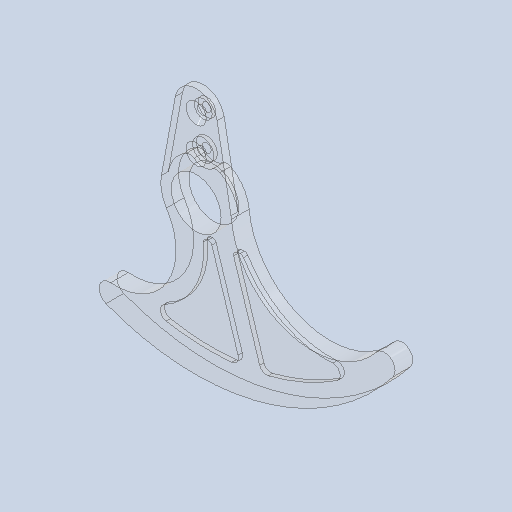
# Autodesk Inventor part: ヘッケン
Saved by Autodesk Inventor 2023 (Build 270158000, 158)
## iProperties
Created: 2022-01-09
Part Number: ヘッケン
Material: ポリカーボネート、クリア
Document SubType Name: Modeling
Designer: acps
Density: 1.2 g/cm^3
Appearance: ポリカーボネート - クリア
Mass: 12.6858 g
Surface Area: 54.0995 cm^2
Volume: 8.90232 cm^3
Author: acps
Autodesk Inventor part; units mm, degrees
ref_plane "YZ Plane" through (0, 0, 0) normal (1, 0, 0) x (0, 1, 0)
ref_plane "XZ Plane" through (0, 0, 0) normal (0, 1, 0) x (-1, 0, 0)
ref_plane "XY Plane" through (0, 0, 0) normal (0, 0, 1) x (1, 0, 0)
sketch "Sketch1" plane through (0, 0, 0) normal (0, 0, 1) x (1, 0, 0)
  line L0 (64.2929, 13) -> (99.1548, 4.0199) construction
  circle A0 centre (64.2929, 13) radius 3 construction
  circle A1 centre (64.2929, 13) radius 4.025 construction
  circle A2 centre (64.2929, 13) radius 7 construction
  arc A3 (102.6474, 8.8986) -> (63.8399, 19.9853) centre (67.7221, -39.8889) ccw construction
  circle A4 centre (99.1548, 4.0199) radius 2.5
  circle A5 centre (99.1548, 4.0199) radius 3.525
  circle A6 centre (99.1548, 4.0199) radius 6
  line L1 (64.2929, 13) -> (98.9408, 0.0186) construction
  line L2 (99.1548, 4.0199) -> (99.1548, -17.9801) construction
  line L3 (99.1548, -17.9801) -> (98.9408, 0.0186) construction
  circle A7 centre (99.1548, -17.9801) radius 10
  circle A8 centre (99.1548, -17.9801) radius 7.025
  line L4 (105.0548, 5.1108) -> (108.9881, -16.162)
  line L5 (93.2548, 5.1108) -> (89.3215, -16.162)
  line L6 (9.3628, -60) -> (214.5663, -60) construction
  arc A9 (95.4028, -0.6623) -> (65.8301, 6.1709) centre (73.5161, -27.9748) ccw construction
  line L7 (99.1548, 4.0199) -> (73.567, -55.2798) construction
  line L8 (99.1548, 4.0199) -> (154.8581, -32.5547) construction
  circle A10 centre (74.7566, -52.523) radius 3
  circle A11 centre (152.3426, -30.903) radius 3
  arc A12 (75.0109, -49.5338) -> (90.7465, -23.3931) centre (76.4523, -32.595) ccw
  arc A13 (109.1059, -16.9921) -> (149.9946, -29.0357) centre (131.9933, -14.7194) ccw
  arc A14 (73.567, -55.2798) -> (154.8581, -32.5547) centre (98.9579, 10.6509) ccw
  circle A15 centre (99.1548, -5.9801) radius 1.25
  circle A16 centre (99.1548, -5.9801) radius 3
  circle A17 centre (99.1548, -5.9801) radius 4.25
  circle A18 centre (99.1548, 4.0199) radius 1.25
  arc A19 (103.9067, -9.1813) -> (101.7399, -9.3536) centre (102.9564, -10.9411) ccw
  arc A20 (96.5698, -9.3536) -> (94.4029, -9.1813) centre (95.3533, -10.9411) ccw
  point P0 (0, 0)
  point P1 (0, 0)
  point P2 (73.6834, -55.3244)
  point P3 (154.7099, -32.7457)
  point P4 (97.1242, -8.1885)
  point P5 (102.5276, -8.5661)
  point P6 (95.7821, -8.5661)
  dimension "d19" = 6
  dimension "d20" = 6
  dimension "d0" = 36
  dimension "d1" = 8.05
  dimension "d2" = 6
  dimension "d3" = 14
  dimension "d4" = 60
  dimension "d5" = 37
  dimension "d6" = 22
  dimension "d7" = 18
  dimension "d8" = 12
  dimension "d9" = 7.05
  dimension "d10" = 20
  dimension "d11" = 14.05
  dimension "d12" = 35
  dimension "d13" = 5
  dimension "d14" = 60
  dimension "d15" = 23.34
  dimension "d17" = 66.6375
  dimension "d18" = 64.5847
  dimension "d21" = 13
  dimension "d23" = 17
  dimension "d29" = 2.5
  dimension "d30" = 6
  dimension "d31" = 8.5
  dimension "d32" = 2.5
  dimension "d43" = 10
  dimension "d44" = 2
  dimension "d45" = 2
  dimension "d46" = 56.711
  dimension "d47" = 23
  constraints: 28 point on circle, 19 centre point, 16 end point, 15 tangent, 11 coincident, 3 point on line, 1 horizontal, 1 vertical, 15 other
  measures "d0" distance of L0.start L0.end
  measures "d1" diameter of A1
  measures "d2" diameter of A0
  measures "d3" diameter of A2
  measures "d4" radius of A3
  measures "d5" distance of L3.end A1.centre
  measures "d6" distance of L2.start L2.end
  measures "d7" distance of L3.end L2.end
  measures "d8" diameter of A6
  measures "d9" diameter of A5
  measures "d10" diameter of A7
  measures "d11" diameter of A8
  measures "d12" radius of A9
  measures "d13" diameter of A4
  measures "d14" distance from line of L6 point (0, 0)
  measures "d15" angle of L2 L7
  measures "d17" distance of L2.start L8.end
  measures "d18" distance of L2.start L7.end
  measures "d21" vertical distance of point (0, 0) L0.start
  measures "d23" radius of A12
  measures "d29" diameter of A15
  measures "d30" diameter of A16
  measures "d31" diameter of A17
  measures "d32" diameter of A18
  measures "d43" distance of A17.centre L0.end
  measures "d44" radius of A19
  measures "d45" radius of A20
  measures "d46" angle of L2 L8
  measures "d47" radius of A13
extrude "Extrusion5" add sketch "Sketch1" against normal blind 5 contours A10 | A7 A20 A17 A19 | A13 A11 A14 A10 A12 A7 | A11
extrude "Extrusion6" add sketch "Sketch1" against normal blind 2 contours A5 | A6 A17 | A6 L4 A7 A17 | A17 A7 A16 A6 | A6 A17 | A6 A17 A7 L5 | A19 A17 A7 | A17 A20 A7 | A7 A16 A17
extrude "Extrusion7" add sketch "Sketch1" against normal blind 3 contours A4 | A16 A7 | A7 A16
chamfer "Chamfer3" distance 1.6 angle 45 2 edges at (97.9048, 4.0199, 0) (97.9048, -5.9801, 0)
sketch "スケッチ5" plane through (0, 0, -5) normal (0, 0, -1) x (-1, 0, 0)
  arc A0 (-149.9946, -29.0357) -> (-154.7099, -32.7457) centre (-152.3426, -30.903) ccw projected
  arc A1 (-154.7099, -32.7457) -> (-73.6834, -55.3244) centre (-98.9579, 10.6509) ccw projected
  arc A2 (-73.6834, -55.3244) -> (-75.0109, -49.5338) centre (-74.7566, -52.523) ccw projected
  arc A3 (-90.7465, -23.3931) -> (-75.0109, -49.5338) centre (-76.4523, -32.595) ccw projected
  arc A4 (-90.7465, -23.3931) -> (-94.4029, -9.1813) centre (-99.1548, -17.9801) ccw projected
  arc A5 (-94.4029, -9.1813) -> (-96.5698, -9.3536) centre (-95.3533, -10.9411) ccw projected
  arc A6 (-101.7399, -9.3536) -> (-96.5698, -9.3536) centre (-99.1548, -5.9801) ccw projected
  arc A7 (-101.7399, -9.3536) -> (-103.9067, -9.1813) centre (-102.9564, -10.9411) ccw projected
  arc A8 (-103.9067, -9.1813) -> (-109.1059, -16.9921) centre (-99.1548, -17.9801) ccw projected
  arc A9 (-149.9946, -29.0357) -> (-109.1059, -16.9921) centre (-131.9933, -14.7194) ccw projected
  circle A10 centre (-99.1548, -17.9801) radius 7.025 projected
  arc A11 (-133.9095, -41.6513) -> (-108.7322, -28.4278) centre (-131.9933, -14.7194) ccw
  arc A12 (-107.7366, -27.9445) -> (-108.7322, -28.4278) centre (-107.8707, -28.9355) ccw
  line L0 (-107.7366, -27.9445) -> (-106.7456, -28.0786)
  arc A13 (-105.9268, -29.3727) -> (-106.7456, -28.0786) centre (-106.8797, -29.0696) ccw
  arc A14 (-149.9946, -29.0357) -> (-109.1059, -16.9921) centre (-131.9933, -14.7194) ccw projected
  line L1 (-125.4948, -36.7823) -> (-91.0171, -41.3623) construction
  arc A15 (-90.7465, -23.3931) -> (-75.0109, -49.5338) centre (-76.4523, -32.595) ccw projected
  line L2 (-125.4948, -36.7823) -> (-99.1548, -17.9801) construction
  line L3 (-99.1548, -17.9801) -> (-91.0171, -41.3623) construction
  line L4 (-99.1548, -17.9801) -> (-114.8496, -67.3215) construction
  line L5 (-105.9268, -29.3727) -> (-113.2937, -52.5329)
  line L6 (-104.7615, -24.3106) -> (-98.127, -25.2082) construction
  arc A16 (-133.9095, -41.6513) -> (-135.1371, -45.326) centre (-134.0514, -43.6463) ccw
  arc A17 (-135.1371, -45.326) -> (-115.702, -53.8625) centre (-98.9579, 10.6509) ccw
  arc A18 (-115.702, -53.8625) -> (-113.2937, -52.5329) centre (-115.1996, -51.9266) ccw
  line L7 (-99.7841, -29.8554) -> (-107.1731, -53.0852)
  arc A19 (-98.697, -29.1675) -> (-99.7841, -29.8554) centre (-98.8311, -30.1585) ccw
  arc A20 (-97.3303, -30.3347) -> (-98.1904, -29.2361) centre (-98.3245, -30.227) ccw
  line L8 (-98.697, -29.1675) -> (-98.1904, -29.2361)
  arc A21 (-97.3303, -30.3347) -> (-86.2751, -51.156) centre (-76.4523, -32.595) ccw
  arc A22 (-86.8471, -54.8905) -> (-86.2751, -51.156) centre (-87.2106, -52.9238) ccw
  arc A23 (-107.1731, -53.0852) -> (-105.4624, -55.6819) centre (-105.2672, -53.6914) ccw
  arc A24 (-105.4624, -55.6819) -> (-86.8471, -54.8905) centre (-98.9579, 10.6509) ccw
  point P0 (0, 0)
  dimension "d57" = 1
  dimension "d58" = 1
  dimension "d59" = 4
  dimension "d60" = 73.669
  dimension "d61" = 36.835
  dimension "d62" = 3
  dimension "d63" = 1
  dimension "d64" = 4
  dimension "d66" = 2
  dimension "d67" = 4
  dimension "d68" = 2
  dimension "d70" = 3
  dimension "d71" = 1
  dimension "d72" = 1
  dimension "d73" = 4
  dimension "d74" = 4
  dimension "d75" = 2
  dimension "d76" = 2
  dimension "d77" = 4
  constraints: 28 point on circle, 18 end point, 17 tangent, 12 centre point, 4 concentric, 4 parallel
  measures "d57" radius of A12
  measures "d58" radius of A13
  measures "d59" radial gap between concentric circles of A11 A9
  measures "d60" angle of L3 L2
  measures "d61" angle of L3 L4
  measures "d62" distance between parallel lines of L4 L5
  measures "d63" distance of L0.start L0.end
  measures "d64" distance between parallel lines of L0 L6
  measures "d66" radius of A16
  measures "d67" radial gap between concentric circles of A1 A17
  measures "d68" radius of A18
  measures "d70" distance between parallel lines of L4 L7
  measures "d71" radius of A19
  measures "d72" radius of A20
  measures "d73" distance between parallel lines of L8 L6
  measures "d74" radial gap between concentric circles of A21 A15
  measures "d75" radius of A22
  measures "d76" radius of A23
  measures "d77" radial gap between concentric circles of A1 A24
extrude "押し出し8" cut sketch "スケッチ5" against normal blind 1.2 contours A11 A12 L0 A13 L5 A18 A17 A16 | A19 L8 A20 A21 A22 A24 A23 L7
body "Solid2"
